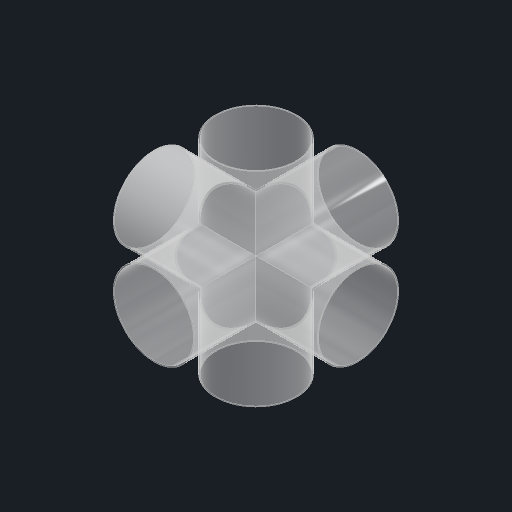
# Autodesk Inventor part: cross
Saved by Autodesk Inventor 2025 (Build 290162000, 162)
## iProperties
Created: 2019-06-03
Part Number: cross
Material: Stainless Steel, Austenitic
Document SubType Name: Modeling
Designer: kuzmin
Density: 8 g/cm^3
Appearance: Polycarbonate - Clear
Mass: 1878.98 g
Surface Area: 3159.79 cm^2
Volume: 234.872 cm^3
Author: kuzmin
Autodesk Inventor part; units mm, degrees
ref_plane "YZ Plane" through (0, 0, 0) normal (1, 0, 0) x (0, 1, 0)
ref_plane "XZ Plane" through (0, 0, 0) normal (0, 1, 0) x (-1, 0, 0)
ref_plane "XY Plane" through (0, 0, 0) normal (0, 0, 1) x (1, 0, 0)
sketch "Sketch1" plane through (0, 0, 0) normal (0, 1, 0) x (-1, 0, 0)
  circle A0 centre (0, 0) radius 51
  dimension "d36" = 102
  constraints: 1 centre point, 1 coincident
  measures "d36" diameter of A0
extrude "Extrusion1" add sketch "Sketch1" along normal mid plane 255.8
pattern_circular "Circular Pattern1" count 2 over 90 about axis through (-10, 0, 0) along (1, 0, 0) of "Extrusion1"
pattern_circular "Circular Pattern2" count 2 over 90 about axis through (0, 0, -10) along (0, 0, 1) of "Extrusion1"
shell "Shell1" thickness 1.5 removed faces 6 at (5.4307, 127.9, 4.7922) at (-15.3374, -12.3475, -127.9) at (-127.9, -13.8083, 6.1282) at (-15.3374, -12.3475, 127.9) at (5.4307, -127.9, 4.7922) at (127.9, -6.8686, 12.0208)
equation "\"d36\" = OD"
equation "\"d2\" = length"
equation "\"d46\" = thickness"
equation "\"OD\" = 102"
equation "\"thickness\" = 1.5"
equation "\"length\" = 255.8"
body "Solid1"
